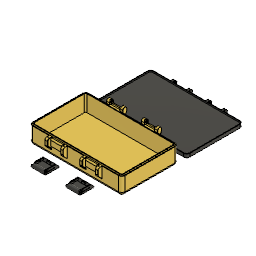
DeWALT Tool Box Double Lock (Autodesk Fusion 360 design; units mm, degrees)
part number: 2025-08-27-12-33-30-467
Autodesk Fusion 360 part; units mm, degrees
note: some values were not read from the file. Chosen so that the rebuilt part matches the saved one: which bodies a step acts on; that a step has no effect; which face or edge a step refers to. Set by a fixed rule: which sketch regions a step uses.
sketch "Box" plane through (0, 0, 0) normal (0, 0, 1) x (1, 0, 0)
  line L0 (65.5, 43) -> (-65.5, 43)
  line L1 (-70.5, 38) -> (-70.5, -38)
  line L2 (-65.5, -43) -> (65.5, -43)
  line L3 (70.5, -38) -> (70.5, 38)
  line L4 (70.5, 43) -> (-70.5, -43) construction
  line L5 (-70.5, 43) -> (70.5, -43) construction
  arc A0 (-65.5, 43) -> (-70.5, 38) centre (-65.5, 38) ccw
  arc A1 (70.5, 38) -> (65.5, 43) centre (65.5, 38) ccw
  arc A2 (65.5, -43) -> (70.5, -38) centre (65.5, -38) ccw
  arc A3 (-70.5, -38) -> (-65.5, -43) centre (-65.5, -38) ccw
  line L6 (65.5, 40) -> (-65.5, 40)
  arc A4 (-65.5, 40) -> (-67.5, 38) centre (-65.5, 38) ccw
  line L7 (-67.5, 38) -> (-67.5, -38)
  arc A5 (-67.5, -38) -> (-65.5, -40) centre (-65.5, -38) ccw
  line L8 (-65.5, -40) -> (65.5, -40)
  arc A6 (65.5, -40) -> (67.5, -38) centre (65.5, -38) ccw
  line L9 (67.5, -38) -> (67.5, 38)
  arc A7 (67.5, 38) -> (65.5, 40) centre (65.5, 38) ccw
  line L10 (-68.5, 38) -> (-68.5, -38)
  arc A8 (-68.5, -38) -> (-65.5, -41) centre (-65.5, -38) ccw
  line L11 (-65.5, -41) -> (65.5, -41)
  arc A9 (65.5, -41) -> (68.5, -38) centre (65.5, -38) ccw
  line L12 (68.5, -38) -> (68.5, 38)
  arc A10 (68.5, 38) -> (65.5, 41) centre (65.5, 38) ccw
  line L13 (65.5, 41) -> (-65.5, 41)
  arc A11 (-65.5, 41) -> (-68.5, 38) centre (-65.5, 38) ccw
  dimension "d5" = 141
  dimension "d6" = 86
  dimension "d7" = 5
  dimension "d10" = -3
  dimension "d95" = 1
  constraint horizontal L0
  constraint perpendicular L0 L1
  constraint parallel L0 L2
  constraint parallel L1 L3
  constraint coincident L4 origin
  constraint coincident L5 origin
  constraint coincident L5.start L0
  constraint coincident L5.start L1
  constraint tangent L0 A0
  constraint tangent L1 A0
  constraint coincident L4.start L0
  constraint coincident L4.start L3
  constraint tangent L0 A1
  constraint tangent L3 A1
  constraint coincident L5.end L3
  constraint coincident L5.end L2
  constraint tangent L3 A2
  constraint tangent L2 A2
  constraint equal A1 A2
  constraint coincident L4.end L2
  constraint coincident L4.end L1
  constraint tangent L2 A3
  constraint tangent L1 A3
  constraint equal A0 A1
  constraint equal A0 A3
  measures "d5" distance of L4.end L5.end
  measures "d6" distance of L5.start L4.end
  measures "d7" radius of A0
extrude "Extrude1" add sketch "Box" along normal blind 26 contours L0 L1 L2 L3 A0 A1 A2 A3 makes body 1
extrude "Extrude15" add sketch "Box" along normal blind 27 contours L10 A8 L11 A9 L12 A10 L13 A11 bodies 1
extrude "Extrude2" add sketch "Box" along normal blind 2 contours L6 A4 L7 A5 L8 A6 L9 A7 bodies 1
chamfer "Chamfer7" distance 0.99 angle 45 8 edges at (0, -41, 26) (-67.6213, -40.1213, 26) (-68.5, 0, 26) (-67.6213, 40.1213, 26) (0, 41, 26) (67.6213, 40.1213, 26) (68.5, 0, 26) (67.6213, -40.1213, 26) on bodies 1
chamfer "Chamfer1" distance 3 angle 45 8 edges at (0, -43, 0) (69.0355, -41.5355, 0) (70.5, 0, 0) (69.0355, 41.5355, 0) (0, 43, 0) (-69.0355, 41.5355, 0) (-70.5, 0, 0) (-69.0355, -41.5355, 0) on bodies 1
fillet "Fillet1" radius 4 8 edges at (-69.0355, 41.5355, 3) (0, 43, 3) (69.0355, 41.5355, 3) (70.5, 0, 3) (69.0355, -41.5355, 3) (0, -43, 3) (-69.0355, -41.5355, 3) (-70.5, 0, 3) on bodies 1
sketch "Lid" plane through (0, 0, 26) normal (0, 0, 1) x (-1, 0, 0)
  arc A0 (70.5, 38) -> (65.5, 43) centre (65.5, 38) ccw
  line L0 (65.5, 43) -> (-65.5, 43)
  arc A1 (-65.5, 43) -> (-70.5, 38) centre (-65.5, 38) ccw
  line L1 (-70.5, 38) -> (-70.5, -38)
  arc A2 (-70.5, -38) -> (-65.5, -43) centre (-65.5, -38) ccw
  line L2 (-65.5, -43) -> (65.5, -43)
  arc A3 (65.5, -43) -> (70.5, -38) centre (65.5, -38) ccw
  line L3 (70.5, -38) -> (70.5, 38)
  arc A4 (65.5, -43) -> (70.5, -38) centre (65.5, -38) ccw
  line L4 (-65.5, -43) -> (65.5, -43)
  line L5 (70.5, -38) -> (70.5, 38)
  arc A5 (70.5, 38) -> (65.5, 43) centre (65.5, 38) ccw
  line L6 (65.5, 43) -> (-65.5, 43)
  arc A6 (-65.5, 43) -> (-70.5, 38) centre (-65.5, 38) ccw
  line L7 (-70.5, 38) -> (-70.5, -38)
  arc A7 (-70.5, -38) -> (-65.5, -43) centre (-65.5, -38) ccw
  line L8 (69.6, -38) -> (69.6, 38)
  arc A8 (69.6, 38) -> (65.5, 42.1) centre (65.5, 38) ccw
  line L9 (65.5, 42.1) -> (-65.5, 42.1)
  arc A9 (-65.5, 42.1) -> (-69.6, 38) centre (-65.5, 38) ccw
  line L10 (-69.6, 38) -> (-69.6, -38)
  arc A10 (-69.6, -38) -> (-65.5, -42.1) centre (-65.5, -38) ccw
  line L11 (-65.5, -42.1) -> (65.5, -42.1)
  arc A11 (65.5, -42.1) -> (69.6, -38) centre (65.5, -38) ccw
  arc A12 (-69.49, -38) -> (-65.5, -41.99) centre (-65.5, -38) ccw
  dimension "d18" = -0.9
extrude "Extrude3" add sketch "Lid" along normal blind 6 separate body contours A0 L0 A1 L1 A2 L2 A3 L3 A4 L4 L5 A5 L6 A6 L7 A7 | L8 A8 L9 A9 L10 A10 L11 A11 makes body 2
extrude "Extrude16" cut sketch "Lid" along normal blind 1 contours L8 A8 L9 A9 L10 A10 L11 A11 bodies 2
chamfer "Chamfer8" distance 1 angle 45 16 edges at (-68.3991, 40.8991, 27) (-69.6, 0, 27) (-68.3991, -40.8991, 27) (0, -42.1, 27) (68.3991, -40.8991, 27) (69.6, 0, 27) (68.3991, 40.8991, 27) (0, 42.1, 27) (0, -43, 32) (69.0355, -41.5355, 32) (70.5, 0, 32) (69.0355, 41.5355, 32) (0, 43, 32) (-69.0355, 41.5355, 32) (-70.5, 0, 32) (-69.0355, -41.5355, 32) on bodies 2
sketch "Lid Hinge and Latch" plane through (0, 0, 0) normal (1, 0, 0) x (0, 1, 0)
  circle A0 centre (46.2, 29) radius 1.8
  line L0 (43, 26) -> (46.2, 26)
  circle A1 centre (-46.2, 29) radius 1.8 construction
  line L1 (-44.8771, 27.5) -> (-43.9639, 27)
  circle A2 centre (-46.2, 29) radius 2
  circle A3 centre (-46.2, 29) radius 3
  line L2 (-44.8771, 30.5) -> (-43.9639, 31)
  line L3 (-49.2, 29) -> (-49.2, 9)
  line L4 (-49.2, 9) -> (-47.7, 9)
  line L5 (-47.7, 9) -> (-43, 13.7)
  line L6 (-43, 13.7) -> (-43, 26.4722)
  line L7 (-46.5, 26.015) -> (-46.5, 15.7)
  line L8 (-46.5, 15.7) -> (-43.5, 15.7)
  line L9 (-46, 15.7) -> (-46, 26.0067)
  line L10 (-43.9639, 27) -> (-43, 26.4722)
  line L11 (-43.5, 15.7) -> (-43, 15.2)
  line L12 (-46.5, 15.7) -> (-43.75, 12.95)
  line L13 (43, 26) -> (43, 31)
  line L14 (-43, 4.6569) -> (-43, 26)
  line L15 (43, 4.6569) -> (43, 26)
  line L16 (-49.2, 29) -> (-49.2, 30.2426)
  line L17 (-49.2, 30.2426) -> (-48.3213, 31.1213)
  line L18 (-38, 0) -> (-40, 0)
  line L19 (42, 32) -> (47, 32)
  line L20 (47, 32) -> (47.6938, 31.6017)
  line L21 (43, 31) -> (42, 32)
  circle A4 centre (46.2, 29) radius 3
  line L22 (-43, 26) -> (-43, 31)
  point P0 (-43, 26.4722)
  point P1 (-38, 0)
  point P2 (42, 32)
  dimension "d37" = 3.6
  dimension "d110" = 3.6
  dimension "d111" = 6
  dimension "d112" = 4
  dimension "d113" = 4
  dimension "d114" = 3
  dimension "d120" = 45
  dimension "d121" = 1.5
  dimension "d124" = 3
  dimension "d130" = 0.5
  dimension "d131" = 2
  dimension "d132" = 45
  dimension "d133" = 0.5
  dimension "d277" = 1.2426
  dimension "d337" = 89.2
  dimension "d342" = 29
  dimension "d343" = 9
  dimension "d353" = 5
  dimension "d354" = 29.863
  dimension "d355" = 6
  dimension "d356" = 89.2
  constraint coincident L1.end A3
  constraint coincident L2.end A3
  constraint concentric A1 A2
  constraint coincident L1.start A2
  constraint coincident A1.centre A2.centre
  constraint coincident L2.start A2
  constraint vertical L1.start L2.start
  constraint vertical L2.end L1.end
  constraint vertical L3
  constraint tangent A3 L3
  constraint perpendicular L3 L4
  constraint perpendicular L4 L6
  constraint vertical L7
  constraint vertical L9
  constraint parallel L1 L10
  constraint coincident A3 L7.start
  constraint coincident A3 L9.end
  constraint horizontal L8
  constraint coincident L9.start L8
  constraint coincident L6 L11.end
  constraint coincident L5 L12.end
  constraint perpendicular L5 L12
  constraint coincident A3 L3.start
  constraint coincident P0 L6.end
  constraint coincident P0 L14
  constraint coincident L0.start L13.start
  constraint perpendicular L0 L13
  constraint parallel L3 L16
  constraint coincident A3 L17.end
  constraint coincident L3.start L16.start
  constraint tangent A3 L17
  constraint horizontal L19
  constraint coincident P2 L19.start
  constraint concentric A0 A4
  constraint coincident L0.end A4
  constraint tangent L0 A4
  constraint coincident L20.end A4
  constraint tangent L20 A4
  measures "d37" diameter of A0
  measures "d110" diameter of A1
  measures "d111" diameter of A3
  measures "d112" distance of L2.end L1.end
  measures "d113" diameter of A2
  measures "d114" distance of L1.start L2.start
  measures "d120" angle of L4 L5
  measures "d121" distance of L3.end L4.end
  measures "d124" distance of L6 L9
  measures "d130" distance of L7.end L9.start
  measures "d131" distance of L5.end L8
  measures "d132" angle of L6 L11
  measures "d133" distance of L6 L8.end
  measures "d277" distance of L3.start L16.end
  measures "d337" distance of A1.centre L15
  measures "d342" distance of A1.centre L18
  measures "d343" distance of L4 L18
  measures "d353" distance of P2 L19.end
  measures "d354" angle of L19 L20
  measures "d355" diameter of A4
  measures "d356" distance of A0.centre L22
extrude "Extrude7" add sketch "Lid Hinge and Latch" along normal mid plane 15 from surface at 26.5 separate body contours L0 L13 L19 L21 A4 | A4 | L19 L20 A4 makes body 3
extrude "Extrude8" add sketch "Lid Hinge and Latch" along normal mid plane 18 from surface at 26.5 contours A0 bodies 3
chamfer "Chamfer2" distance 0.5 angle 45 2 faces at (17.5, 46.1024, 28.7514) (35.5, 46.1024, 28.7514) on bodies 3
sketch "Lid Hinge Cut" plane through (0, 43, 0) normal (0, 1, 0) x (-1, 0, 0)
  line L0 (-65.5, 26) -> (65.5, 26)
  line L1 (65.5, 26) -> (65.5, 31)
  line L2 (-65.5, 31) -> (-65.5, 26)
  line L3 (-34, 30.8) -> (-35.5, 29.934) construction
  line L4 (-35.5, 29.934) -> (-35.5, 30.8) construction
  line L5 (-35.5, 30.8) -> (-34, 30.8) construction
  line L6 (-19, 30.8) -> (-17.5, 29.934) construction
  line L7 (-17.5, 29.934) -> (-17.5, 30.8) construction
  line L8 (-17.5, 30.8) -> (-19, 30.8) construction
  line L9 (-35, 30.8) -> (-35, 27.2)
  line L10 (-18, 27.2) -> (-18, 30.8)
  line L11 (-35.5, 27.7) -> (-35.5, 30.3)
  line L12 (-17.5, 30.3) -> (-17.5, 27.7)
  line L13 (65.5, 31) -> (-65.5, 31)
  line L14 (-19, 26) -> (-19, 31)
  line L15 (-34, 31) -> (-34, 26)
  line L16 (-29, 32) -> (-24, 32)
  line L17 (-24, 32) -> (-24, 26)
  line L18 (-24, 26) -> (-29, 26)
  line L19 (-29, 26) -> (-29, 32)
  line L20 (-19, 32) -> (-34, 32)
  dimension "d357" = 30
  dimension "d358" = 30
  dimension "d365" = 5
  dimension "d366" = 5
  constraint perpendicular L0 L4
  constraint perpendicular L4 L5
  constraint perpendicular L0 L7
  constraint perpendicular L7 L8
  constraint coincident L3.end L11
  constraint coincident L6.end L12
  constraint coincident L3.start L15
  constraint coincident L6.start L14
  constraint coincident L5 L9.start
  constraint coincident L8 L10.end
  constraint horizontal L16
  constraint vertical L17
  constraint horizontal L18
  constraint vertical L19
  constraint coincident L0 L17.end
  constraint coincident L16.start L20
  measures "d357" angle of L3 L5
  measures "d358" angle of L6 L8
  measures "d365" distance of L17 L20.start
  measures "d366" distance of L16.start L20.end
extrude "Extrude40" cut sketch "Lid Hinge Cut" along normal through all contours L0 L13 L17 L18 L19 | L13 L16 L17 L19 L20 bodies 3
extrude "Extrude26" add sketch "Lid Hinge and Latch" along normal mid plane 20 from surface at 26.5 separate body contours L1 A2 A3 L2 | A3 L6 L8 L9 L10 L11 L14 L22 | A3 L3 L4 L5 L7 L12 | L5 L6 L8 L11 L12 L14 | A3 L16 L17 picked at (-44.3747, 30.9359) makes body 4
extrude "Extrude27" add sketch "Lid Hinge and Latch" along normal mid plane 17 from surface at 26.5 contours A2 bodies 4
extrude "Extrude28" add sketch "Lid Hinge and Latch" along normal mid plane 18 from surface at 26.5 contours L1 A2 A3 L2 | L1 A2 A3 L2 bodies 4
chamfer "Chamfer14" distance 0.49 angle 45 2 edges at (35, -48.0647, 29.7232) (18, -48.0647, 29.7232) on bodies 4
chamfer "Chamfer15" distance 0.5 angle 45 2 edges at (35.5, -43.2, 29) (17.5, -43.2, 29) on bodies 4
extrude "Extrude29" cut sketch "Lid Hinge and Latch" along normal mid plane 17 from surface at 26.5 contours A3 L6 L8 L9 L10 L11 L14 L22 | L5 L6 L8 L11 L12 L14 bodies 4
extrude "Extrude30" add sketch "Lid Hinge and Latch" along normal mid plane 5 from surface at 26.5 contours L5 L6 L8 L11 L12 L14 bodies 4
chamfer "Chamfer18" distance 0.4 angle 45 3 edges at (35, -43, 20.0861) (18, -43, 20.0861) (26.5, -49.2, 9) on bodies 4
fillet "Fillet4" radius 1 1 edges at (26.5, -47.7, 9) on bodies 4
sketch "Box and Lacth Hinge" plane through (0, 0, 0) normal (1, 0, 0) x (0, 1, 0)
  line L0 (43, 26) -> (43, 18)
  line L1 (-46.2, 32) -> (-42, 32)
  line L2 (-46, 24) -> (-46, 16.2)
  line L3 (-45.5, 15.7) -> (-43, 15.7)
  line L4 (-43, 9) -> (-43, 26)
  line L5 (-46, 16.2) -> (-45.5, 15.7)
  arc A0 (-46.2, 26) -> (-49.2, 23) centre (-46.2, 23) ccw
  line L6 (-49.2, 23) -> (-49.2, 16.8569)
  line L7 (-48.0284, 14.0284) -> (-43, 9)
  line L8 (-45.5, 15.7) -> (-43, 13.2)
  line L9 (43.2, 26) -> (43.2, 29)
  line L10 (48.0284, 23.0284) -> (43, 18)
  arc A1 (-49.2, 16.8569) -> (-48.0284, 14.0284) centre (-45.2, 16.8569) ccw
  circle A2 centre (-46.2, 29) radius 3
  line L11 (-43, 26) -> (-46.2, 26)
  arc A3 (-44, 26) -> (-46, 24) centre (-44, 24) ccw
  line L12 (43, 26) -> (45.0864, 26)
  line L13 (-43, 26) -> (-43, 31)
  circle A4 centre (-46.2, 29) radius 1.8
  arc A5 (48.0284, 23.0284) -> (49.2, 25.8569) centre (45.2, 25.8569) ccw
  line L14 (49.2, 29) -> (49.2, 25.8569)
  circle A6 centre (46.2, 29) radius 2
  circle A7 centre (46.2, 29) radius 1.8 construction
  circle A8 centre (46.2, 29) radius 3
  line L15 (47.7, 30.3229) -> (48.2, 31.2361)
  line L16 (44.7, 30.3229) -> (44.2, 31.2361)
  circle A9 centre (46.2, 29) radius 3.2 construction
  line L17 (43, 26) -> (46.2, 26)
  line L18 (-38, 0) -> (38, 0)
  line L19 (-43, 31) -> (-42, 32)
  line L20 (-46.2, 32) -> (-47, 32)
  line L21 (-47, 32) -> (-47.6938, 31.6017)
  circle A10 centre (46.2, 29) radius 1.3
  line L22 (47.3136, 26) -> (49.2, 26)
  arc A11 (45.0864, 26) -> (47.3136, 26) centre (46.2, 29) ccw
  point P0 (-46, 15.7)
  point P1 (-46, 15.7)
  point P2 (-49.2, 29)
  point P3 (-48.8, 9)
  point P4 (43, 26)
  point P5 (43, 26)
  point P6 (43, 31)
  dimension "d136" = 0.5
  dimension "d137" = 0.5
  dimension "d140" = 3
  dimension "d150" = 45
  dimension "d182" = 45
  dimension "d239" = 4
  dimension "d244" = 3
  dimension "d252" = 2
  dimension "d270" = 4
  dimension "d309" = 3.6
  dimension "d310" = 6
  dimension "d311" = 4
  dimension "d312" = 4
  dimension "d313" = 3
  dimension "d321" = 6.4
  dimension "d352" = 18
  dimension "d363" = 0.8
  constraint vertical L2
  constraint horizontal L3
  constraint vertical L4
  constraint coincident P1 L2
  constraint coincident P1 L3
  constraint horizontal A0.end A0.centre
  constraint vertical L6
  constraint parallel L5 L8
  constraint coincident L4 L3.end
  constraint vertical L9
  constraint coincident L0.end L10.end
  constraint vertical L0
  constraint tangent L6 A1
  constraint tangent L7 A1
  constraint coincident A2 A0.start
  constraint tangent A2 L11
  constraint horizontal L11
  constraint coincident L11 A3.start
  constraint tangent L2 A3
  constraint tangent L11 A3
  constraint coincident P1 P0
  constraint coincident L4 L8.end
  constraint vertical A0.end P2
  constraint coincident L1.start A2
  constraint horizontal L1
  constraint horizontal L4.start P3
  constraint horizontal L12
  constraint coincident P5 P4
  constraint coincident L12 A11.start
  constraint tangent L10 A5
  constraint vertical L14
  constraint coincident A5.end L14.end
  constraint tangent A5 L14
  constraint coincident L15.end A8
  constraint coincident L16.end A8
  constraint concentric A6 A7
  constraint coincident L15.start A6
  constraint coincident L16.start A6
  constraint coincident L9.end A8
  constraint horizontal L9.end A6.centre
  constraint coincident L14.start A8
  constraint concentric A8 A9
  constraint horizontal L14.start A6.centre
  constraint horizontal L15.start L16.start
  constraint horizontal L16.end L15.end
  constraint vertical L1.start A2.centre
  constraint coincident A6.centre A7.centre
  constraint coincident L12 L9.start
  constraint tangent A2 L20
  constraint coincident A2 L21.end
  constraint tangent A2 L21
  constraint coincident L1.end L19.end
  constraint coincident L12.end A9
  constraint coincident A9 L22.start
  constraint coincident L14 L22.end
  constraint perpendicular L14 L22
  constraint horizontal L12.end L22.start
  constraint concentric A9 A11
  measures "d136" distance of P1 L2.end
  measures "d137" distance of P1 L3.start
  measures "d140" distance of L2 L4
  measures "d150" angle of L4 L7
  measures "d182" angle of L0 L10
  measures "d239" radius of A1
  measures "d244" radius of A0
  measures "d252" radius of A3
  measures "d270" radius of A5
  measures "d309" diameter of A7
  measures "d310" diameter of A8
  measures "d311" distance of L16.end L15.end
  measures "d312" diameter of A6
  measures "d313" distance of L15.start L16.start
  measures "d321" diameter of A9
  measures "d352" distance of L0.end L18
  measures "d363" distance of L1.start L20.end
extrude "Extrude11" add sketch "Box and Lacth Hinge" along normal mid plane 25 from surface at 26.5 separate body contours L0 L10 L12 A5 L14 L17 L22 A11 | L9 L12 A8 L17 | A6 A8 L15 L16 | L14 A8 L17 L22 A11 | A6 A8 L15 L16 | A6 | A10 makes body 5
extrude "Extrude10" cut sketch "Box and Lacth Hinge" along normal mid plane 15.4 from surface at 26.5 contours L9 L12 A8 L17 | A6 A8 L15 L16 | L14 A8 L17 L22 A11 | A6 A8 L15 L16 | L1 A2 L11 L13 L19 bodies 5
extrude "Extrude12" cut sketch "Box and Lacth Hinge" along normal mid plane 18.4 from surface at 26.5 contours A6 | A10 bodies 5
extrude "Extrude39" cut sketch "Box and Lacth Hinge" along normal mid plane 17.4 from surface at 26.5 contours A6 A8 L15 L16 picked at (44.5493, 31.0867) bodies 5
chamfer "Chamfer4" distance 0.499 angle 45 2 faces at (17.3, 47.1704, 28.4739) (35.7, 46.3483, 28.35) on bodies 5
chamfer "Chamfer21" distance 0.5 distance2 0.5 2 edges at (17.8, 46.2, 32) (35.2, 46.2, 32) measured on face at (15.6, 43.8719, 30.892) measured on face at (37.4, 48.5281, 30.892) on bodies 5
chamfer "Chamfer3" distance 0.2 angle 45 10 edges at (14, 46.2, 32) (14, 49.2, 27.4284) (14, 48.8955, 24.3261) (14, 45.5142, 20.5142) (14, 43.2, 27.5) (39, 49.2, 27.4284) (39, 46.2, 32) (39, 43.2, 27.5) (39, 45.5142, 20.5142) (39, 48.8955, 24.3261) on bodies 5
extrude "Extrude31" add sketch "Box and Lacth Hinge" along normal mid plane 28 from surface at 26.5 separate body contours L1 A2 L11 L13 L19 | A2 | A2 L20 L21 | A4 makes body 6
extrude "Extrude32" cut sketch "Box and Lacth Hinge" along normal mid plane 20.4 from surface at 26.5 contours L1 A2 L11 L13 L19 | A2 | A2 L20 L21 bodies 6
extrude "Extrude33" cut sketch "Box and Lacth Hinge" along normal mid plane 17.4 from surface at 26.5 contours A4 bodies 6 makes body 7 at (40.5, -45.1333, 29.6667)
chamfer "Chamfer17" distance 0.5 angle 45 2 edges at (35.2, -47.8782, 28.3491) (17.8, -47.8782, 29.6509) on bodies 6 7
chamfer "Chamfer16" distance 0.2 angle 45 6 edges at (40.5, -49.0987, 28.227) (40.5, -47.3469, 31.8008) (40.5, -44.6, 26) (12.5, -49.0987, 28.227) (12.5, -44.6, 26) (12.5, -47.3469, 31.8008) on bodies 6 7
extrude "Extrude21" add sketch "Box and Lacth Hinge" along normal mid plane 28 from surface at 26.5 separate body contours L2 L4 L5 A0 L6 L7 L8 A1 L11 A3 | L2 L3 L4 L5 L11 A3 | L3 L4 L8 makes body 8
extrude "Extrude22" cut sketch "Box and Lacth Hinge" along normal mid plane 20.4 from surface at 26.5 contours L2 L4 L5 A0 L6 L7 L8 A1 L11 A3 | L2 L3 L4 L5 L11 A3 | L3 L4 L8 bodies 8 makes body 9 at (40.5, -44.6761, 16.3428)
chamfer "Chamfer11" distance 0.2 angle 45 10 edges at (12.5, -49.2, 19.9284) (12.5, -48.3213, 25.1213) (12.5, -44.6, 26) (12.5, -45.5142, 11.5142) (12.5, -48.8955, 15.3261) (40.5, -49.2, 19.9284) (40.5, -48.8955, 15.3261) (40.5, -45.5142, 11.5142) (40.5, -44.6, 26) (40.5, -48.3213, 25.1213) on bodies 8 9
sketch "Latch Side" plane through (0, 0, 0) normal (1, 0, 0) x (0, 1, 0)
  line L0 (-48.0284, 14.0284) -> (-43, 9)
  line L1 (-43, 9) -> (-43, 26)
  arc A0 (-46.2, 26) -> (-49.2, 23) centre (-46.2, 23) ccw
  line L2 (-49.2, 23) -> (-49.2, 16.8569)
  arc A1 (-49.2, 16.8569) -> (-48.0284, 14.0284) centre (-45.2, 16.8569) ccw
  line L3 (-43, 26) -> (-46.2, 26)
  line L4 (-43, 25) -> (-46.2, 25)
  arc A2 (-46.2, 25) -> (-48.2, 23) centre (-46.2, 23) ccw
  line L5 (-48.2, 23) -> (-48.2, 16.8569)
  arc A3 (-48.2, 16.8569) -> (-47.3213, 14.7355) centre (-45.2, 16.8569) ccw
  line L6 (-47.3213, 14.7355) -> (-43, 10.4142)
  dimension "d224" = -1
  constraint coincident L1 L6.end
  constraint coincident L1 L4.start
extrude "Extrude25" cut sketch "Latch Side" along normal mid plane 21.4 from surface at 26.5 contours L1 L4 A2 L5 A3 L6 bodies 8 9
chamfer "Chamfer13" distance 0.49 angle 45 10 edges at (15.8, -44.6, 25) (15.8, -45.1607, 12.5749) (15.8, -47.9716, 15.7088) (15.8, -48.2, 19.9284) (15.8, -47.6142, 24.4142) (37.2, -47.6142, 24.4142) (37.2, -48.2, 19.9284) (37.2, -47.9716, 15.7088) (37.2, -45.1607, 12.5749) (37.2, -44.6, 25) on bodies 8 9
extrude "Extrude19" add sketch "Box and Lacth Hinge" along normal mid plane 16.6 from surface at 26.5 separate body contours L2 L3 L4 L5 L11 A3 | L3 L4 L8 makes body 10
extrude "Extrude20" cut sketch "Box and Lacth Hinge" along normal mid plane 5.6 from surface at 26.5 contours L3 L4 L8 bodies 10
ref_plane "WorkPlane1" through (26.5, -44.5, 19.6) normal (0, 1, 0) x (0, 0, 1)
sketch "Nub" plane through (0, -44.5, 0) normal (0, 1, 0) x (1, 0, 0)
  line L0 (18.2, -20.1) -> (34.8, -20.1)
  line L1 (18.2, -16.2) -> (18.2, -24)
  line L2 (34.8, -24) -> (34.8, -16.2)
  line L3 (18.2, -20.1) -> (17.6, -20.1)
  line L4 (18.6, -21.1) -> (34.4, -21.1)
  line L5 (34.8, -20.1) -> (35.4, -20.1)
  line L6 (17.6, -20.1) -> (35.4, -20.1)
  arc A0 (17.6, -20.1) -> (18.6, -21.1) centre (18.6, -20.1) ccw
  arc A1 (34.4, -21.1) -> (35.4, -20.1) centre (34.4, -20.1) ccw
  arc A2 (17.485, -20.1) -> (18.6, -21.215) centre (18.6, -20.1) ccw
  line L7 (18.6, -21.215) -> (34.4, -21.215)
  arc A3 (34.4, -21.215) -> (35.515, -20.1) centre (34.4, -20.1) ccw
  line L8 (17.485, -20.1) -> (17.6, -20.1)
  line L9 (35.4, -20.1) -> (35.515, -20.1)
  point P0 (26.5, -20.1)
  dimension "d176" = 1
  dimension "d225" = 16.6
  dimension "d226" = 17.8
  dimension "d228" = 1
  dimension "d229" = 1
  dimension "d231" = 0.115
  constraint horizontal L0
  constraint coincident L0.end L2
  constraint midpoint L0.start L1
  constraint perpendicular L1 L3
  constraint perpendicular L2 L4
  constraint horizontal L5
  constraint equal L3 L5
  constraint midpoint L0 P0
  constraint midpoint P0 L6
  constraint tangent L4 A0
  constraint coincident L3.end L6.start
  constraint tangent L4 A1
  constraint parallel L3 L8
  constraint parallel L5 L9
  measures "d176" distance of L0 L4
  measures "d225" distance of L0.start L0.end
  measures "d226" distance of L3.end L5.end
  measures "d228" radius of A0
  measures "d229" radius of A1
revolve "Revolve1" add sketch "Nub" angle 360 about axis through (18.2, -44.5, 20.1) along (1, 0, 0) contours L0 L1 L2 L4 L6 A0 A1 | L1 L3 L6 A0 | L2 L5 L6 A1 bodies 10
revolve "Revolve2" cut sketch "Nub" angle 360 about axis through (18.2, -44.5, 20.1) along (1, 0, 0) contours L1 L3 L6 A0 | L2 L5 L6 A1 | L1 A0 A2 L8 | L2 A1 A3 L9 bodies 4
mirror "Mirror8" about plane through (0, 0, 0) normal (1, 0, 0) of bodies 7 6 8 9 4 3 5 10 makes body 11 at (-30.6, 43, 23.3333) makes body 12 at (-20.6667, 44, 32) makes body 13 at (-12.5, -44.629, 16.4176) makes body 14 at (-40.5, -44.629, 16.4176) makes body 15 at (-12.5, -45.1333, 29.7333) makes body 16 at (-25.5667, -43, 22.5667) makes body 17 at (-40.5, -45.1333, 29.7333) makes body 18 at (-29.5, -49.2, 15.9333)
combine "Combine8" operation add target body 2 tool bodies 6 7 15 17 12 3
combine "Combine9" operation add target body 1 tool bodies 14 13 8 9 5 11 16 10
sketch "Column Divider" plane through (0, 0, 2) normal (0, 0, 1) x (-1, 0, 0)
  arc A0 (-67.5, -38) -> (-65.5, -40) centre (-65.5, -38) ccw
  line L0 (-65.5, -40) -> (65.5, -40)
  arc A1 (65.5, -40) -> (67.5, -38) centre (65.5, -38) ccw
  line L1 (67.5, -38) -> (67.5, 38)
  arc A2 (67.5, 38) -> (65.5, 40) centre (65.5, 38) ccw
  line L2 (65.5, 40) -> (-65.5, 40)
  arc A3 (-65.5, 40) -> (-67.5, 38) centre (-65.5, 38) ccw
  line L3 (-67.5, 38) -> (-67.5, -38)
  line L4 (68.5, -41) -> (68.5, 41)
  line L5 (67.5, 1) -> (69.5, 1)
  line L6 (69.5, 1) -> (69.5, -1)
  line L7 (69.5, -1) -> (67.5, -1)
  line L8 (67.5, -1) -> (67.5, 1)
  line L9 (67.5, 1) -> (69.5, -1) construction
  line L10 (69.5, 1) -> (67.5, -1) construction
  point P0 (65.5, 41)
  point P1 (68.5, 38)
  point P2 (65.5, -41)
  point P3 (68.5, -38)
  point P4 (68.5, 0)
  dimension "d344" = 2
  dimension "d345" = 2
  constraint vertical L4
  constraint horizontal L4.start P2
  constraint horizontal L4.end P0
  constraint coincident L4 P1
  constraint horizontal L5
  constraint perpendicular L5 L6
  constraint parallel L5 L7
  constraint parallel L6 L8
  constraint coincident L9 P4
  constraint coincident L10 P4
  constraint midpoint L4 P4
  measures "d344" distance of L6.end L7.end
  measures "d345" distance of L5.end L6.end
extrude "Extrude35" add sketch "Column Divider" along normal blind 25 thin wall 2 centred separate body open curves L4 makes body 19
extrude "Extrude41" add sketch "Column Divider" against normal blind 2 contours L1 L4 L5 L7 L8 | L4 L5 L6 L7 bodies 19
pattern_linear "R-Pattern1" [no effect]
delete_body "RemoveBody1" bodies 19
sketch "Row Divider" plane through (0, 0, 2) normal (0, 0, 1) x (-1, 0, 0)
  arc A0 (-67.5, -38) -> (-65.5, -40) centre (-65.5, -38) ccw
  line L0 (-65.5, -40) -> (65.5, -40)
  arc A1 (65.5, -40) -> (67.5, -38) centre (65.5, -38) ccw
  line L1 (67.5, -38) -> (67.5, 38)
  arc A2 (67.5, 38) -> (65.5, 40) centre (65.5, 38) ccw
  line L2 (65.5, 40) -> (-65.5, 40)
  arc A3 (-65.5, 40) -> (-67.5, 38) centre (-65.5, 38) ccw
  line L3 (-67.5, 38) -> (-67.5, -38)
  line L4 (68.5, 41) -> (-68.5, 41)
  line L5 (-1, 42) -> (1, 42)
  line L6 (1, 42) -> (1, 40)
  line L7 (1, 40) -> (-1, 40)
  line L8 (-1, 40) -> (-1, 42)
  line L9 (-1, 42) -> (1, 40) construction
  line L10 (1, 42) -> (-1, 40) construction
  point P0 (65.5, 41)
  point P1 (68.5, 38)
  point P2 (-68.5, 38)
  point P3 (0, 41)
  dimension "d348" = 2
  dimension "d349" = 2
  constraint horizontal L4
  constraint coincident L4 P0
  constraint vertical L4.start P1
  constraint vertical L4.end P2
  constraint horizontal L5
  constraint perpendicular L5 L6
  constraint parallel L5 L7
  constraint parallel L6 L8
  constraint coincident L9 P3
  constraint coincident L10 P3
  constraint midpoint L4 P3
  measures "d348" distance of L6.end L7.end
  measures "d349" distance of L5.end L6.end
extrude "Extrude36" add sketch "Row Divider" along normal blind 25 thin wall 2 centred separate body open curves L4 makes body 20
extrude "Extrude42" add sketch "Row Divider" against normal blind 2 contours L2 L4 L6 L7 L8 | L4 L5 L6 L8 bodies 20
pattern_linear "R-Pattern2" [no effect]
delete_body "RemoveBody2" bodies 20
sketch "DeWALT Logo" plane through (0, 0, 32) normal (0, 0, 1) x (-1, 0, 0)
  line L0 (-40.5, 42) -> (-65.5, 42)
  arc A0 (-65.5, 42) -> (-69.5, 38) centre (-65.5, 38) ccw
  line L1 (-69.5, 38) -> (-69.5, -38)
  arc A1 (-69.5, -38) -> (-65.5, -42) centre (-65.5, -38) ccw
  line L2 (-65.5, -42) -> (-34, -42)
  line L3 (-34, -42) -> (-34, -47)
  line L4 (-34, -47) -> (-29, -47)
  line L5 (-29, -47) -> (-29, -43)
  line L6 (-29, -43) -> (-24, -43)
  line L7 (-24, -43) -> (-24, -47)
  line L8 (-24, -47) -> (-19, -47)
  line L9 (-19, -47) -> (-19, -42)
  line L10 (-19, -42) -> (19, -42)
  line L11 (19, -42) -> (19, -47)
  line L12 (19, -47) -> (24, -47)
  line L13 (24, -47) -> (24, -43)
  line L14 (24, -43) -> (29, -43)
  line L15 (29, -43) -> (29, -47)
  line L16 (29, -47) -> (34, -47)
  line L17 (34, -47) -> (34, -42)
  line L18 (34, -42) -> (65.5, -42)
  arc A2 (65.5, -42) -> (69.5, -38) centre (65.5, -38) ccw
  line L19 (69.5, -38) -> (69.5, 38)
  arc A3 (69.5, 38) -> (65.5, 42) centre (65.5, 38) ccw
  line L20 (65.5, 42) -> (40.5, 42)
  line L21 (40.5, 42) -> (40.5, 46.5983)
  line L22 (40.5, 46.5983) -> (40.3, 47)
  line L23 (40.3, 47) -> (36.7, 47)
  line L24 (36.7, 47) -> (36.7, 42)
  line L25 (36.7, 42) -> (16.3, 42)
  line L26 (16.3, 42) -> (16.3, 47)
  line L27 (16.3, 47) -> (12.7, 47)
  line L28 (12.7, 47) -> (12.5, 46.5983)
  line L29 (12.5, 46.5983) -> (12.5, 42)
  line L30 (12.5, 42) -> (-12.5, 42)
  line L31 (-12.5, 42) -> (-12.5, 46.5983)
  line L32 (-12.5, 46.5983) -> (-12.7, 47)
  line L33 (-12.7, 47) -> (-16.3, 47)
  line L34 (-16.3, 47) -> (-16.3, 42)
  line L35 (-16.3, 42) -> (-36.7, 42)
  line L36 (-36.7, 42) -> (-36.7, 47)
  line L37 (-36.7, 47) -> (-40.3, 47)
  line L38 (-40.3, 47) -> (-40.5, 46.5983)
  line L39 (-40.5, 46.5983) -> (-40.5, 42)
  line L40 (-37.5, 43) -> (37.5, 43) construction
  line L41 (37.5, 43) -> (37.5, -43) construction
  line L42 (37.5, -43) -> (-37.5, -43) construction
  line L43 (-37.5, -43) -> (-37.5, 43) construction
  line L44 (-37.5, 43) -> (37.5, -43) construction
  line L45 (37.5, 43) -> (-37.5, -43) construction
  line L46 (37.5028, -9.0615) -> (-37.5414, -9.0615)
  line L47 (-37.5414, -9.0615) -> (-37.5414, -7.6387)
  line L48 (-37.5414, -7.6387) -> (37.5028, -7.6387)
  line L49 (37.5028, -7.6387) -> (37.5028, -9.0615)
  line L50 (37.5028, 7.6636) -> (-37.5387, 7.6636)
  line L51 (-37.5387, 7.6636) -> (-37.5387, 9.0857)
  line L52 (-37.5387, 9.0857) -> (37.5028, 9.0857)
  line L53 (37.5028, 9.0857) -> (37.5028, 7.6636)
  line L54 (-26.1569, -6.9254) -> (-37.5424, -6.9254)
  line L55 (-37.5424, -6.9254) -> (-37.5424, -3.0095)
  line L56 (-37.5424, -3.0095) -> (-34.4561, -3.0095)
  line L57 (-34.4561, -3.0095) -> (-34.4561, 6.9207)
  line L58 (-34.4561, 6.9207) -> (-29.2314, 6.9207)
  line L59 (-29.2314, 6.9207) -> (-29.2314, -3.0095)
  line L60 (-29.2314, -3.0095) -> (-26.1569, -3.0095)
  line L61 (-26.1569, -3.0095) -> (-26.1569, -6.9254)
  line L62 (-18.3273, -6.9254) -> (-18.3273, 6.9207)
  line L63 (-18.3273, 6.9207) -> (-27.8146, 6.9207)
  line L64 (-27.8146, 6.9207) -> (-27.8146, 2.7942)
  line L65 (-27.8146, 2.7942) -> (-23.5441, 2.7942)
  line L66 (-23.5441, 2.7942) -> (-23.5441, -6.9254)
  line L67 (-23.5441, -6.9254) -> (-18.3273, -6.9254)
  line L68 (-13.3747, -6.9277) -> (-7.6434, -6.9277)
  line L69 (-7.6434, -6.9277) -> (-3.135, 6.9207)
  line L70 (-3.135, 6.9207) -> (-8.4641, 6.9207)
  line L71 (-8.4641, 6.9207) -> (-8.9396, 4.8133)
  line L72 (-8.9396, 4.8133) -> (-12.1406, 4.8133)
  line L73 (-12.1406, 4.8133) -> (-12.6637, 6.9207)
  line L74 (-12.6637, 6.9207) -> (-17.7684, 6.9207)
  line L75 (-17.7684, 6.9207) -> (-13.3747, -6.9277)
  line L76 (-9.6516, 1.7325) -> (-10.5611, -2.2997)
  line L77 (-10.5611, -2.2997) -> (-11.4295, 1.7325)
  line L78 (-11.4295, 1.7325) -> (-9.6516, 1.7325)
  line L79 (-4.8922, -6.9277) -> (0.207, -6.9277)
  line L80 (0.207, -6.9277) -> (1.6297, -0.1666)
  line L81 (1.6297, -0.1666) -> (3.1727, -6.9277)
  line L82 (3.1727, -6.9277) -> (7.6804, -6.9277)
  line L83 (7.6804, -6.9277) -> (9.1343, -0.1666)
  line L84 (9.1343, -0.1666) -> (10.5262, -6.9277)
  line L85 (10.5262, -6.9277) -> (15.6191, -6.9277)
  line L86 (15.6191, -6.9277) -> (11.8122, 6.9207)
  line L87 (11.8122, 6.9207) -> (7.0844, 6.9207)
  line L88 (7.0844, 6.9207) -> (5.4941, 0.1636)
  line L89 (5.4941, 0.1636) -> (3.8627, 6.9207)
  line L90 (3.8627, 6.9207) -> (-0.9795, 6.9207)
  line L91 (-0.9795, 6.9207) -> (-4.8922, -6.9277)
  line L92 (23.1264, -3.9623) -> (15.5304, -3.9623)
  line L93 (15.5304, -3.9623) -> (15.5304, -1.1126)
  line L94 (15.5304, -1.1126) -> (19.2068, -1.1126)
  line L95 (19.2068, -1.1126) -> (19.2068, 0.07)
  line L96 (19.2068, 0.07) -> (16.0058, 0.07)
  line L97 (16.0058, 0.07) -> (16.0058, 2.9203)
  line L98 (16.0058, 2.9203) -> (19.2068, 2.9203)
  line L99 (19.2068, 2.9203) -> (19.2068, 4.1022)
  line L100 (19.2068, 4.1022) -> (15.5307, 4.1022)
  line L101 (15.5307, 4.1022) -> (15.5307, 6.9207)
  line L102 (15.5307, 6.9207) -> (23.1264, 6.9207)
  line L103 (23.1264, 6.9207) -> (23.1264, -3.9623)
  line L104 (31.0125, -6.9277) -> (37.4992, -6.9277)
  line L105 (37.4992, -6.9277) -> (37.4992, 6.9207)
  line L106 (37.4992, 6.9207) -> (31.0371, 6.9207)
  spline S0 degree 3 poles (31.0371, 6.9207) (27.0844, 6.9207) (24.1351, 4.7607) (24.1351, 0.0249) knots 0 0 0 0 1 1 1 1
  spline S1 degree 3 poles (24.1351, 0.0249) (24.1351, -4.7108) (27.1813, -6.9274) (31.0125, -6.9277) knots 0 0 0 0 1 1 1 1
  line L107 (32.1444, 2.7738) -> (32.5535, 2.7738)
  line L108 (32.5535, 2.7738) -> (32.5535, -2.9474)
  line L109 (32.5535, -2.9474) -> (32.1339, -2.9474)
  spline S2 degree 3 poles (32.1339, -2.9474) (30.4914, -2.9474) (29.4153, -2.3309) (29.4153, -0.0207) knots 0 0 0 0 1 1 1 1
  spline S3 degree 3 poles (29.4153, -0.0207) (29.4153, 2.0835) (30.5009, 2.7738) (32.1444, 2.7738) knots 0 0 0 0 1 1 1 1
  point P0 (-65.5, -43)
  point P1 (-65.5, 43)
  dimension "d437" = 75
  constraint horizontal L40
  constraint perpendicular L40 L41
  constraint parallel L40 L42
  constraint horizontal L42.end P0
  constraint coincident origin L45
  constraint horizontal L40.start P1
  measures "d437" distance of L41 L43
extrude "Extrude43" add sketch "DeWALT Logo" against normal blind 0.6 separate body contours L46 L47 L48 L49 | L50 L51 L52 L53 | L54 L55 L56 L57 L58 L59 L60 L61 | L62 L63 L64 L65 L66 L67 | L68 L69 L70 L71 L72 L73 L74 L75 | L79 L80 L81 L82 L83 L84 L85 L86 L87 L88 L89 L90 L91 | L92 L93 L94 L95 L96 L97 L98 L99 L100 L101 L102 L103 | L104 L105 L106 S0 S1 makes body 21 at (20.0662, -0.9298, 32) makes body 22 at (-35.8507, -0.9223, 32) makes body 23 at (-21.8198, -1.0095, 32) makes body 24 at (32.7145, -3.6107, 32) makes body 25 at (6.81, -0.5752, 32) makes body 26 at (12.5266, 8.113, 32) makes body 27 at (-12.1885, 0.0579, 32) makes body 28 at (12.5249, -8.1377, 32)
scale "Scale1" factor 1 about (0, 0, 32) bodies 21 23 24 25 26 27 28 22
combine "Combine10" operation cut target body 2 tool bodies 21 23 24 25 26 27 28 22 keep tools
move_body "Move4" bodies 4 18 to x (1, 0, 0) y (0, 0, 1) z (0, -1, 0) at (0, -17.2, 75.2)
move_body "Move5" bodies 4 18 to x (1, 0, 0) y (0, 1, 0) z (0, 0, 1) at (0, -25, -26)
move_body "Move8" bodies 2 21 22 23 24 25 26 27 28 to x (1, 0, 0) y (0, -1, 0) z (0, 0, -1) at (0, 84, 64)
move_body "Move7" bodies 2 21 22 23 24 25 26 27 28 to x (1, 0, 0) y (0, 1, 0) z (0, 0, 1) at (0, 15, -32)
sketch "Insert" plane through (0, 0, 2) normal (0, 0, 1) x (-1, 0, 0)
  arc A0 (-67.5, -38) -> (-65.5, -40) centre (-65.5, -38) ccw
  line L0 (-65.5, -40) -> (65.5, -40)
  arc A1 (65.5, -40) -> (67.5, -38) centre (65.5, -38) ccw
  line L1 (67.5, -38) -> (67.5, 38)
  arc A2 (67.5, 38) -> (65.5, 40) centre (65.5, 38) ccw
  line L2 (65.5, 40) -> (-65.5, 40)
  arc A3 (-65.5, 40) -> (-67.5, 38) centre (-65.5, 38) ccw
  line L3 (-67.5, 38) -> (-67.5, -38)
  line L4 (67.3, -38) -> (67.3, 38)
  arc A4 (67.3, 38) -> (65.5, 39.8) centre (65.5, 38) ccw
  line L5 (65.5, 39.8) -> (-65.5, 39.8)
  arc A5 (-65.5, 39.8) -> (-67.3, 38) centre (-65.5, 38) ccw
  line L6 (-67.3, 38) -> (-67.3, -38)
  arc A6 (-67.3, -38) -> (-65.5, -39.8) centre (-65.5, -38) ccw
  line L7 (-65.5, -39.8) -> (65.5, -39.8)
  arc A7 (65.5, -39.8) -> (67.3, -38) centre (65.5, -38) ccw
  dimension "d379" = -0.2
extrude "Extrude45" [rolled back] along distance 15 taper angle 0
sketch "Sketch22" plane through (0, 0, 17) normal (0, 0, 1) x (-1, 0, 0)
  arc A0 (65.5, -39.8) -> (67.3, -38) centre (65.5, -38) ccw
  line L0 (67.3, -38) -> (67.3, 38)
  arc A1 (67.3, 38) -> (65.5, 39.8) centre (65.5, 38) ccw
  line L1 (65.5, 39.8) -> (-65.5, 39.8)
  arc A2 (-65.5, 39.8) -> (-67.3, 38) centre (-65.5, 38) ccw
  line L2 (-67.3, 38) -> (-67.3, -38)
  arc A3 (-67.3, -38) -> (-65.5, -39.8) centre (-65.5, -38) ccw
  line L3 (-65.5, -39.8) -> (65.5, -39.8)
  line L4 (67.3, 0) -> (-67.3, 0)
  line L5 (67.3, -13.3333) -> (-67.3, -13.3333) construction
  line L6 (-67.3, 13.3333) -> (67.3, 13.3333) construction
  line L7 (65.5, -40) -> (-65.5, -40)
  line L8 (-65.5, 40) -> (65.5, 40)
  line L9 (-62.9, 9.65) -> (62.9, 9.65) construction
  line L10 (62.9, 9.65) -> (62.9, -9.65) construction
  line L11 (62.9, -9.65) -> (-62.9, -9.65) construction
  line L12 (-62.9, -9.65) -> (-62.9, 9.65) construction
  line L13 (-62.9, 9.65) -> (62.9, -9.65) construction
  line L14 (62.9, 9.65) -> (-62.9, -9.65) construction
  line L15 (-26.4, -9.65) -> (-26.4, 9.65) construction
  line L16 (57.2, -9.65) -> (57.2, 9.65) construction
  line L17 (42.7, -9.65) -> (42.7, 9.65) construction
  line L18 (62.9, 0) -> (57.2, 0)
  line L19 (57.2, 0) -> (57.2, -4) construction
  line L20 (57.7, -4) -> (62.4, -4)
  line L21 (62.9, -3.5) -> (62.9, 0)
  line L22 (57.2, -4.5) -> (57.2, -6.65)
  line L23 (57.2, -6.65) -> (54.396, -9.368)
  line L24 (53.4214, -9.6104) -> (42.7, -6.5)
  arc A4 (53.4214, -9.6104) -> (54.396, -9.368) centre (53.7, -8.65) ccw
  line L25 (32.2, -9.65) -> (32.2, 9.65) construction
  line L26 (42.7, -6.5) -> (32.2, -6.5)
  line L27 (32.2, -6.5) -> (29.7, -7)
  line L28 (29.7, -7) -> (-0.3, -7)
  line L29 (-7.3, -9.65) -> (-7.3, 9.65) construction
  line L30 (-25.4, -6.35) -> (-7.3, -6.35)
  line L31 (-0.3, -7) -> (-7.3, -6.35)
  line L32 (-26.8726, -3.9741) -> (-62.4274, -2.0259)
  line L33 (-26.4, -4.4734) -> (-26.4, -5.35)
  arc A5 (-26.4, -5.35) -> (-25.4, -6.35) centre (-25.4, -5.35) ccw
  line L34 (-62.9, -1.5266) -> (-62.9, 0)
  arc A6 (-62.9, -1.5266) -> (-62.4274, -2.0259) centre (-62.4, -1.5266) ccw
  arc A7 (57.7, -4) -> (57.2, -4.5) centre (57.7, -4.5) ccw
  line L35 (62.4, -4) -> (62.9, -3.5)
  line L36 (63.4, -3.7071) -> (63.4, 0)
  line L37 (62.6071, -4.5) -> (63.4, -3.7071)
  line L38 (58, -4.5) -> (62.6071, -4.5)
  line L39 (57.7, -4.8) -> (57.7, -6.8617)
  line L40 (57.7, -6.8617) -> (54.744, -9.727)
  arc A8 (53.2818, -10.0905) -> (54.744, -9.727) centre (53.7, -8.65) ccw
  line L41 (53.2818, -10.0905) -> (42.6289, -7)
  line L42 (42.6289, -7) -> (32.2495, -7)
  line L43 (32.2495, -7) -> (29.7495, -7.5)
  line L44 (29.7495, -7.5) -> (-0.3227, -7.5)
  line L45 (-0.3227, -7.5) -> (-7.3227, -6.85)
  line L46 (-25.3943, -6.85) -> (-7.3227, -6.85)
  arc A9 (-26.9, -5.35) -> (-25.3943, -6.85) centre (-25.4, -5.35) ccw
  line L47 (-26.9, -4.7574) -> (-26.9, -5.35)
  line L48 (-27.1836, -4.4578) -> (-62.4547, -2.5251)
  arc A10 (-63.4, -1.5266) -> (-62.4547, -2.5251) centre (-62.4, -1.5266) ccw
  line L49 (-63.4, -1.5266) -> (-63.4, 0)
  arc A11 (58, -4.5) -> (57.7, -4.8) centre (58, -4.8) ccw
  arc A12 (-26.4, -4.4734) -> (-26.8726, -3.9741) centre (-26.9, -4.4734) ccw
  arc A13 (-26.9, -4.7574) -> (-27.1836, -4.4578) centre (-27.2, -4.7574) ccw
  point P0 (62.9, -4)
  point P1 (-26.4, -4)
  point P2 (-62.9, -2)
  dimension "d387" = 125.8
  dimension "d388" = 19.3
  dimension "d389" = 36.5
  dimension "d390" = 5.7
  dimension "d391" = 14.5
  dimension "d392" = 69.1
  dimension "d393" = 4
  dimension "d394" = 3
  dimension "d395" = 6.65
  dimension "d397" = 6.5
  dimension "d398" = 3.5
  dimension "d399" = 1
  dimension "d400" = 10.5
  dimension "d401" = 7
  dimension "d402" = 2.5
  dimension "d403" = 30
  dimension "d404" = 7
  dimension "d405" = 6.35
  dimension "d406" = 4
  dimension "d407" = 1
  dimension "d408" = 2
  dimension "d409" = 0.5
  dimension "d412" = 0.5
  dimension "d413" = 0.5
  dimension "d414" = 0.5
  dimension "d415" = 0.3
  dimension "d416" = 0.5
  dimension "d417" = 0.3
  dimension "d418" = 26.6667
  dimension "d419" = 26.6667
  constraint midpoint L0 L4.start
  constraint midpoint L2 L4.end
  constraint coincident L0 L5.start
  constraint coincident L2 L5.end
  constraint perpendicular L2 L5
  constraint coincident L2 L6.start
  constraint coincident L0 L6.end
  constraint perpendicular L0 L6
  constraint horizontal L9
  constraint perpendicular L9 L10
  constraint parallel L9 L11
  constraint parallel L10 L12
  constraint coincident L13 origin
  constraint coincident L14 origin
  constraint coincident L11 L15.start
  constraint coincident L9 L15.end
  constraint perpendicular L9 L15
  constraint coincident L11 L16.start
  constraint coincident L9 L16.end
  constraint perpendicular L9 L16
  constraint coincident L11 L17.start
  constraint coincident L9 L17.end
  constraint perpendicular L9 L17
  constraint horizontal L18
  constraint vertical L19
  constraint horizontal L20
  constraint vertical L21
  constraint coincident L16 L19.end
  constraint midpoint L10 L18.start
  constraint coincident L16 L22.end
  constraint coincident L17 L24.end
  constraint tangent L23 A4
  constraint tangent L24 A4
  constraint tangent L11 A4
  constraint coincident L11 L25.start
  constraint coincident L9 L25.end
  constraint perpendicular L9 L25
  constraint coincident L25 L26.end
  constraint perpendicular L25 L26
  constraint perpendicular L25 L28
  constraint coincident L11 L29.start
  constraint coincident L9 L29.end
  constraint perpendicular L9 L29
  constraint coincident L29 L30.end
  constraint perpendicular L29 L30
  constraint coincident L15 P1
  constraint coincident L12 P2
  constraint tangent L30 A5
  constraint tangent L33 A5
  constraint vertical L33
  constraint midpoint L12 L34.end
  constraint coincident P2 L32
  constraint coincident P2 L34
  constraint tangent L32 A6
  constraint tangent L34 A6
  constraint coincident L19.end L22
  constraint coincident L19.end L20
  constraint tangent L22 A7
  constraint tangent L20 A7
  constraint coincident P0 L20
  constraint coincident P0 L21
  constraint concentric A4 A8
  constraint concentric A5 A9
  constraint concentric A6 A10
  constraint tangent A10 L49
  constraint tangent L48 A10
  constraint tangent L40 A8
  constraint tangent L38 A11
  constraint tangent L39 A11
  constraint coincident P1 L32
  constraint coincident P1 L33
  constraint tangent L32 A12
  constraint tangent L33 A12
  constraint tangent L47 A13
  constraint tangent L48 A13
  measures "d387" distance of L10.end L11.end
  measures "d388" distance of L9.end L10.end
  measures "d389" distance of L12 L15
  measures "d390" distance of L10 L16
  measures "d391" distance of L16 L17
  measures "d392" distance of L15 L17
  measures "d393" distance of L18.end L19.end
  measures "d394" distance of L16.start L22.end
  measures "d395" distance of L18.end L22.end
  measures "d397" distance of L4 L24.end
  measures "d398" distance of L16 A4.centre
  measures "d399" radius of A4
  measures "d400" distance of L17 L25
  measures "d401" distance of L4 L28
  measures "d402" horizontal distance of L26.end L27.end
  measures "d403" distance of L27.end L28.end
  measures "d404" distance of L28.end L29
  measures "d405" distance of L4 L30
  measures "d406" distance of L4 P1
  measures "d407" radius of A5
  measures "d408" distance of L4 P2
  measures "d409" radius of A6
  measures "d412" radius of A7
  measures "d413" distance of P0 L20.end
  measures "d414" distance of P0 L21.start
  measures "d415" radius of A11
  measures "d416" radius of A12
  measures "d417" radius of A13
  measures "d418" distance of L5 L7
  measures "d419" distance of L6 L8
revolve "Revolve3" [rolled back] along angle 360
pattern_linear "R-Pattern3" [rolled back] u space distance 25 v space distance 0
pattern_linear "R-Pattern4" [rolled back] u space distance -25 v space distance 0
sketch "Sketch23" plane through (0, 0, 17) normal (0, 0, 1) x (-1, 0, 0)
  line L0 (-61.8, 36) -> (-35.8, 36)
  line L1 (-33.8, 34) -> (-33.8, -34)
  line L2 (-35.8, -36) -> (-61.8, -36)
  line L3 (-63.8, -34) -> (-63.8, 34)
  line L4 (-63.8, 36) -> (-33.8, -36) construction
  line L5 (-33.8, 36) -> (-63.8, -36) construction
  line L6 (-67.3, 38) -> (-67.3, -38)
  arc A0 (-35.8, -36) -> (-33.8, -34) centre (-35.8, -34) ccw
  arc A1 (-63.8, -34) -> (-61.8, -36) centre (-61.8, -34) ccw
  arc A2 (-33.8, 34) -> (-35.8, 36) centre (-35.8, 34) ccw
  arc A3 (-61.8, 36) -> (-63.8, 34) centre (-61.8, 34) ccw
  point P0 (-48.8, 0)
  dimension "d428" = 30
  dimension "d429" = 72
  dimension "d430" = 3.5
  dimension "d431" = 2
  constraint horizontal L0
  constraint perpendicular L0 L1
  constraint parallel L0 L2
  constraint parallel L1 L3
  constraint coincident L4 P0
  constraint coincident L5 P0
  constraint horizontal origin P0
  constraint coincident L4.end L1
  constraint coincident L4.end L2
  constraint tangent L1 A0
  constraint tangent L2 A0
  constraint coincident L5.end L3
  constraint coincident L5.end L2
  constraint tangent L3 A1
  constraint tangent L2 A1
  constraint equal A0 A1
  constraint coincident L5.start L1
  constraint coincident L5.start L0
  constraint tangent L1 A2
  constraint tangent L0 A2
  constraint equal A0 A2
  constraint coincident L4.start L3
  constraint coincident L4.start L0
  constraint tangent L3 A3
  constraint tangent L0 A3
  constraint equal A0 A3
  measures "d428" distance of L4.end L5.end
  measures "d429" distance of L5.start L4.end
  measures "d430" distance of L3 L6
  measures "d431" radius of A0
extrude "Extrude46" [rolled back] along distance -10 taper angle 0
chamfer "Chamfer22" [rolled back] distance 1
chamfer "Chamfer23" [rolled back] distance 0.5
equation "Width = ( ( SlotWidth + 2 mm ) * Rows ) + 4 mm"
equation "Length = ( ( SlotLength + 2 mm ) * Columns ) + 4 mm"
equation "Height = SlotHeight + 8 mm"
equation "ConrnerRadius = 5 mm"
equation "d5 = Length"
equation "d6 = Width"
equation "d7 = ConrnerRadius"
equation "d11 = Height - 7 mm"
equation "HingePosition = ( HingesDistance / 2 ) + 14 mm"
equation "d46 = HingePosition"
equation "d47 = HingeSize"
equation "d49 = HingePosition"
equation "d50 = HingeSize + 3 mm"
equation "d61 = HingePosition"
equation "d62 = HingeSize + 0.4 mm"
equation "d64 = HingePosition"
equation "d65 = HingeSize + 10 mm"
equation "d67 = HingePosition"
equation "d68 = HingeSize + 3.4 mm"
equation "HingesDistance = ( Length - ( ConrnerRadius * 2 ) - 56 mm ) / 3"
equation "d97 = Height - 6 mm"
equation "d147 = HingePosition"
equation "d148 = LatchSize - 3.4 mm"
equation "d152 = HingePosition"
equation "d155 = HingePosition"
equation "d156 = LatchSize + 8 mm"
equation "d158 = HingePosition"
equation "d159 = LatchSize + 0.4 mm"
equation "d171 = HingePosition"
equation "d172 = LatchSize + 1.4 mm"
equation "HingeSize = 15 mm"
equation "LatchSize = 20 mm"
equation "d187 = HingePosition"
equation "d188 = LatchSize"
equation "d190 = HingePosition"
equation "d191 = LatchSize - 3 mm"
equation "d193 = HingePosition"
equation "d194 = LatchSize - 2 mm"
equation "d198 = HingePosition"
equation "d199 = LatchSize - 3 mm"
equation "d201 = HingePosition"
equation "d209 = HingePosition"
equation "d210 = LatchSize + 8 mm"
equation "d212 = HingePosition"
equation "d213 = LatchSize + 0.4 mm"
equation "d215 = HingePosition"
equation "d216 = LatchSize - 2.6 mm"
equation "d226 = LatchSize - 2.2 mm"
equation "d257 = -Height + 7 mm"
equation "d261 = -Height + 1 mm"
equation "d279 = Height - 8 mm"
equation "RowSectionDistance = ( Width - 4 mm ) / Rows"
equation "ColumnSectionDistance = ( Length - 4 mm ) / Columns"
equation "d283 = Columns"
equation "d285 = ColumnSectionDistance"
equation "d288 = Height - 8 mm"
equation "d290 = Rows"
equation "d292 = RowSectionDistance"
equation "Rows = 1"
equation "Columns = 1"
equation "d324 = HingePosition"
equation "d325 = HingeSize + 2.4 mm"
equation "d337 = Width + 3.2 mm"
equation "SlotWidth = 80 mm"
equation "SlotLength = 135 mm"
equation "SlotHeight = 25 mm"
equation "d342 = Height - 4 mm"
equation "d343 = Height - 24 mm"
equation "d352 = Height - 15 mm"
equation "d356 = Width + 3.2 mm"
equation "d393 = ( 8 / 2 ) * 1 mm"
equation "d397 = ( 13 / 2 ) * 1 mm"
equation "d401 = ( 14 / 2 ) * 1 mm"
equation "d405 = ( 12.7 / 2 ) * 1 mm"
equation "d406 = ( 8 / 2 ) * 1 mm"
equation "d408 = ( 4 / 2 ) * 1 mm"
equation "d414 = d413"
equation "d418 = SlotWidth / 3"
equation "d419 = SlotWidth / 3"
equation "LogoWidth = 75 mm"
equation "d437 = LogoWidth"
equation "d438 = LogoWidth / 75 mm"
named bodies: "Box", "Lid", "Body8 (1)", "Body9 (1)", "Body12 (1)", "Body14 (1)", "Body16 (1)", "Body18 (1)", "Body20 (1)", "Body25 (1)", "Body27 (1)", "Body29 (1)", "Body30 (1)", "Body30 (2)", "Body31 (1)", "Body31 (1) (1)", "Latch 1", "Lid Hinge", "Latch 2"
